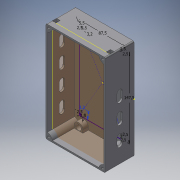
# Autodesk Inventor part: Base caixa principal
Saved by Autodesk Inventor 2019 (Build 230136000, 136)
## iProperties
Created: 2020-06-01
Part Number: Base caixa principal
Material: Generic
Document SubType Name: Modeling
Designer: luiza
Density: 1 g/cm^3
Appearance: Default
Author: luiza
Autodesk Inventor part; units mm, degrees
ref_plane "YZ Plane" through (0, 0, 0) normal (1, 0, 0) x (0, 1, 0)
ref_plane "XZ Plane" through (0, 0, 0) normal (0, 1, 0) x (-1, 0, 0)
ref_plane "XY Plane" through (0, 0, 0) normal (0, 0, 1) x (1, 0, 0)
sketch "Sketch1" plane through (0, 0, 0) normal (0, 0, 1) x (1, 0, 0)
  line L0 (-55, -92.5) -> (55, -92.5)
  line L1 (55, -92.5) -> (55, 92.5)
  line L2 (55, 92.5) -> (-55, 92.5)
  line L3 (-55, 92.5) -> (-55, -92.5)
  line L4 (-55, -92.5) -> (55, 92.5) construction
  line L5 (55, -92.5) -> (-55, 92.5) construction
  point P0 (0, 0)
  dimension "d0" = 185
  dimension "d1" = 110
  constraints: 12 end point, 2 midpoint, 2 parallel, 1 horizontal, 1 perpendicular
  measures "d0" distance of L0.end L1.end
  measures "d1" distance of L1.end L2.end
extrude "Extrusion1" add sketch "Sketch1" along normal blind 3
sketch "Sketch10" plane through (0, 0, 3) normal (0, 0, 1) x (1, 0, 0)
  line L0 (-43.75, -73.75) -> (43.75, -73.75)
  line L1 (43.75, -73.75) -> (43.75, 73.75)
  line L2 (43.75, 73.75) -> (-43.75, 73.75)
  line L3 (-43.75, 73.75) -> (-43.75, -73.75)
  line L4 (-43.75, -73.75) -> (43.75, 73.75) construction
  line L5 (43.75, -73.75) -> (-43.75, 73.75) construction
  point P0 (0, 0)
  dimension "d51" = 87.5
  dimension "d52" = 147.5
  constraints: 12 end point, 2 midpoint, 2 parallel, 1 horizontal, 1 perpendicular
  measures "d51" distance of L2.end L1.end
  measures "d52" distance of L1.end L0.end
sketch "Sketch2" plane through (0, 0, 3) normal (0, 0, 1) x (1, 0, 0)
  line L0 (-55, -92.5) -> (55, -92.5) projected
  line L1 (55, -92.5) -> (55, 92.5) projected
  line L2 (55, 92.5) -> (-55, 92.5) projected
  line L3 (-55, 92.5) -> (-55, -92.5) projected
  line L4 (56.6239, 0) -> (-62.9531, 0)
  line L5 (0, -95.1843) -> (0, 95.8224)
  line L6 (-42.8653, -89.5) -> (42.8653, -89.5)
  line L7 (52, -80.3653) -> (52, 80.3653)
  line L8 (55, 92.5) -> (-55, 92.5) projected
  arc A0 (-52, 80.3653) -> (-42.8653, 89.5) centre (-55, 92.5) ccw
  line L9 (42.8653, 89.5) -> (-42.8653, 89.5)
  line L10 (-52, 80.3653) -> (-52, -80.3653)
  arc A1 (-42.8653, -89.5) -> (-52, -80.3653) centre (-55, -92.5) ccw
  arc A2 (42.8653, 89.5) -> (52, 80.3653) centre (55, 92.5) ccw
  arc A3 (52, -80.3653) -> (42.8653, -89.5) centre (55, -92.5) ccw
  point P0 (0, 0)
  constraints: 12 end point, 9 symmetric about line, 8 point on circle, 4 centre point, 1 coincident, 1 horizontal, 1 vertical, 3 other
extrude "Extrusion2" add sketch "Sketch2" along normal blind 50 contours L3 L4 L10 A1 L6 L5 L0 | L5 L6 A3 L7 L4 L1 L0 | L3 L2 L5 L9 A0 L10 L4 | L4 L7 A2 L9 L5 L2 L1
sketch "Sketch3" plane through (0, 0, 53) normal (0, 0, 1) x (1, 0, 0)
  arc A0 (-52, 80.3653) -> (-42.8653, 89.5) centre (-55, 92.5) ccw projected
  line L0 (-42.8653, 89.5) -> (42.8653, 89.5) projected
  arc A1 (42.8653, 89.5) -> (52, 80.3653) centre (55, 92.5) ccw projected
  line L1 (52, 80.3653) -> (52, -80.3653) projected
  arc A2 (52, -80.3653) -> (42.8653, -89.5) centre (55, -92.5) ccw projected
  line L2 (42.8653, -89.5) -> (-42.8653, -89.5) projected
  arc A3 (-42.8653, -89.5) -> (-52, -80.3653) centre (-55, -92.5) ccw projected
  line L3 (-52, -80.3653) -> (-52, 80.3653) projected
  line L4 (-55, -92.5) -> (55, -92.5) projected
  line L5 (55, -92.5) -> (55, 92.5) projected
  line L6 (55, 92.5) -> (-55, 92.5) projected
  line L7 (-55, 92.5) -> (-55, -92.5) projected
  circle A4 centre (50, 87.5) radius 2.01
  line L8 (-58.744, 0) -> (58.8874, 0)
  circle A5 centre (50, -87.5) radius 2.01
  circle A6 centre (-50, 87.5) radius 2.01
  circle A7 centre (-50, -87.5) radius 2.01
  point P0 (0, 0)
  dimension "d17" = 5
  dimension "d18" = 5
  dimension "d22" = 4.02
  dimension "d57" = 5
  dimension "d58" = 5
  dimension "d59" = 5
  dimension "d60" = 5
  dimension "d61" = 5
  constraints: 4 centre point, 2 end point, 1 horizontal, 1 symmetric about line, 1 other
  measures "d17" distance from line of L5 A4.centre
  measures "d18" distance from line of L6 A4.centre
  measures "d22" diameter of A4
  measures "d57" distance from line of L7 A6.centre
  measures "d58" distance from line of L6 A6.centre
  measures "d59" distance from line of L4 A7.centre
  measures "d60" distance from line of L7 A7.centre
  measures "d61" distance from line of L4 A5.centre
extrude "Extrusion3" cut sketch "Sketch3" against normal blind 24 contours A4 | A5 | A6 | A7
ref_plane "Work Plane1" through (0, 0, 43) normal (0, 0, 1) x (1, 0, 0)
sketch "Sketch5" plane through (0, 0, 43) normal (0, 0, 1) x (1, 0, 0)
  circle A0 centre (-50, 87.5) radius 2.01 projected
  line L0 (-46.49, 92.5) -> (-46.49, 85.4735)
  line L1 (-46.49, 85.4735) -> (-50, 83.447)
  line L2 (-50, 83.447) -> (-53.51, 85.4735)
  line L3 (-53.51, 85.4735) -> (-53.51, 92.5)
  line L4 (-53.51, 89.5265) -> (-50, 91.553) construction
  line L5 (-50, 91.553) -> (-46.49, 89.5265) construction
  line L6 (55, 92.5) -> (-55, 92.5) projected
  line L7 (-46.49, 92.5) -> (-53.51, 92.5)
  line L8 (0, 97.1182) -> (0, -98.0167)
  line L9 (52.0686, 0) -> (-60.1376, 0)
  circle A1 centre (-50, -87.5) radius 2.01
  line L10 (-46.49, -92.5) -> (-46.49, -85.4735)
  line L11 (-46.49, -85.4735) -> (-50, -83.447)
  line L12 (-50, -83.447) -> (-53.51, -85.4735)
  line L13 (-53.51, -85.4735) -> (-53.51, -92.5)
  line L14 (-53.51, -89.5265) -> (-50, -91.553) construction
  line L15 (-50, -91.553) -> (-46.49, -89.5265) construction
  line L16 (-46.49, -92.5) -> (-53.51, -92.5)
  line L17 (46.49, 92.5) -> (46.49, 85.4735)
  line L18 (46.49, 85.4735) -> (50, 83.447)
  line L19 (50, 83.447) -> (53.51, 85.4735)
  line L20 (53.51, 85.4735) -> (53.51, 92.5)
  line L21 (53.51, 89.5265) -> (50, 91.553) construction
  line L22 (50, 91.553) -> (46.49, 89.5265) construction
  line L23 (46.49, 92.5) -> (53.51, 92.5)
  circle A2 centre (50, -87.5) radius 2.01
  line L24 (46.49, -92.5) -> (46.49, -85.4735)
  line L25 (46.49, -85.4735) -> (50, -83.447)
  line L26 (50, -83.447) -> (53.51, -85.4735)
  line L27 (53.51, -85.4735) -> (53.51, -92.5)
  line L28 (53.51, -89.5265) -> (50, -91.553) construction
  line L29 (50, -91.553) -> (46.49, -89.5265) construction
  line L30 (46.49, -92.5) -> (53.51, -92.5)
  line L31 (-42.8653, 89.5) -> (42.8653, 89.5) projected
  line L32 (55, -92.5) -> (55, 92.5) projected
  circle A3 centre (50, 87.5) radius 2.01 projected
  point P0 (0, 0)
  point P1 (-46.49, 87.5)
  point P2 (-46.49, -87.5)
  point P3 (46.49, 87.5)
  point P4 (46.49, -87.5)
  dimension "d54" = 7.02
  dimension "d55" = 7.02
  dimension "d56" = 7.02
  dimension "d62" = 5
  constraints: 60 end point, 29 symmetric about line, 14 point on line, 3 parallel, 2 centre point, 2 horizontal, 2 vertical, 1 equal length, 1 horizontal alignment, 1 vertical alignment, 2 other
  measures "d54" distance between parallel lines of L3 L0
  measures "d55" distance between parallel lines of L5 L2
  measures "d56" distance between parallel lines of L4 L1
  measures "d62" distance from line of L32 L18.end
extrude "Extrusion4" cut sketch "Sketch5" against normal blind 8 contours L0 L1 L2 L3 L6 | L20 L19 L18 L17 L6 | L16 L13 L12 L11 L10 | L24 L25 L26 L27 L30 | A3
fillet "Fillet1" radius 2 4 edges at (-55, 92.5, 26.5) (55, 92.5, 26.5) (-55, -92.5, 26.5) (55, -92.5, 26.5)
sketch "Sketch11" plane through (0, 0, 3) normal (0, 0, 1) x (1, 0, 0)
  circle A0 centre (-34.7653, 84.1) radius 3.01
  line L0 (-42.8653, 89.5) -> (42.8653, 89.5) projected
  circle A1 centre (-34.7653, 84.1) radius 5.1 construction
  circle A2 centre (-34.7653, 84.1) radius 8.1 construction
  line L1 (-58.7196, 0) -> (55.3155, 0)
  line L2 (0, 98.8118) -> (0, -110.7956)
  circle A3 centre (-34.7653, -84.1) radius 3.01
  circle A4 centre (34.7653, 84.1) radius 3.01
  circle A5 centre (34.7653, -84.1) radius 3.01
  arc A6 (-52, 80.3653) -> (-42.8653, 89.5) centre (-55, 92.5) ccw projected
  line L3 (-42.8653, 89.5) -> (-42.8653, 76) construction
  point P0 (0, 0)
  dimension "d63" = 6.02
  dimension "d64" = 5.4
  dimension "d65" = 10.2
  dimension "d66" = 3
  constraints: 6 centre point, 6 end point, 3 symmetric about line, 2 vertical, 1 coincident, 1 horizontal, 1 tangent, 3 other
  measures "d63" diameter of A0
  measures "d64" distance from line of L0 A0.centre
  measures "d65" diameter of A1
  measures "d66" radial gap between concentric circles of A1 A2
extrude "Extrusion7" cut sketch "Sketch11" against normal blind 3
sketch "Sketch12" plane through (0, 0, 3) normal (0, 0, 1) x (1, 0, 0)
  circle A0 centre (-34.7653, 84.1) radius 3.01 projected
  circle A1 centre (-34.7653, 84.1) radius 5.1
  arc A2 (-42.8653, 84.1) -> (-26.6653, 84.1) centre (-34.7653, 84.1) ccw
  line L0 (-26.6653, 84.1) -> (-26.6653, 92.5)
  line L1 (53, 92.5) -> (-53, 92.5) projected
  line L2 (-26.6653, 92.5) -> (-42.8653, 92.5)
  line L3 (-54.2433, 0) -> (61.8693, 0)
  line L4 (0, -98.8908) -> (0, 99.1403)
  circle A3 centre (-34.7653, -84.1) radius 5.1
  arc A4 (-26.6653, -84.1) -> (-42.8653, -84.1) centre (-34.7653, -84.1) ccw
  line L5 (-26.6653, -84.1) -> (-26.6653, -92.5)
  line L6 (-26.6653, -92.5) -> (-42.8653, -92.5)
  line L7 (-53, -92.5) -> (53, -92.5) projected
  circle A5 centre (34.7653, 84.1) radius 3.01
  circle A6 centre (34.7653, 84.1) radius 5.1
  arc A7 (26.6653, 84.1) -> (42.8653, 84.1) centre (34.7653, 84.1) ccw
  line L8 (26.6653, 84.1) -> (26.6653, 92.5)
  line L9 (26.6653, 92.5) -> (42.8653, 92.5)
  circle A8 centre (34.7653, -84.1) radius 5.1
  arc A9 (42.8653, -84.1) -> (26.6653, -84.1) centre (34.7653, -84.1) ccw
  line L10 (26.6653, -84.1) -> (26.6653, -92.5)
  line L11 (0, -92.5) -> (42.8653, -92.5)
  line L12 (42.8653, 89.5) -> (-42.8653, 89.5) projected
  line L13 (-52, -80.3653) -> (-52, 80.3653) projected
  line L14 (-42.8653, 84.1) -> (-42.8653, 92.5)
  line L15 (42.8653, 84.1) -> (42.8653, 96.4532)
  line L16 (-42.8653, -84.1) -> (-42.8653, -92.5)
  line L17 (42.8653, -84.1) -> (42.8653, -92.5)
  point P0 (0, 0)
  point P1 (-40.9253, 89.3597)
  point P2 (-40.9253, 92.5)
  point P3 (-40.9253, -92.5)
  point P4 (40.9253, 92.5)
  point P5 (40.9253, -92.5)
  dimension "d70" = 10.2
  dimension "d71" = 3
  constraints: 28 end point, 13 symmetric about line, 11 point on line, 9 centre point, 8 point on circle, 6 vertical, 2 coincident, 1 collinear, 1 horizontal, 7 other
  measures "d70" diameter of A1
  measures "d71" radial gap between concentric circles of A1 A2
extrude "Extrusion8" add sketch "Sketch12" along normal blind 10 contours L14 L12 L0 A2 | L14 L1 L0 L12 | L12 L15 A7 L8 | L8 L1 L15 L12 | L5 L6 L16 A4 | L10 A9 L17 L7
sketch "Sketch13" plane through (0, 0, 3) normal (0, 0, 1) x (1, 0, 0)
  line L0 (43.75, 73.75) -> (-43.75, 73.75) construction
  line L1 (43.75, -73.75) -> (43.75, 73.75) construction
  line L2 (-43.75, 73.75) -> (-43.75, -73.75) construction
  line L3 (-43.75, -73.75) -> (43.75, -73.75) construction
  circle A0 centre (-41.25, 71.25) radius 1.6
  line L4 (-43.4734, 71.25) -> (-34.0393, 71.25)
  line L5 (-44.5409, 71.25) -> (-42.8954, 68.4) construction
  line L6 (-42.8954, 68.4) -> (-39.6046, 68.4) construction
  line L7 (-39.6046, 68.4) -> (-37.9591, 71.25) construction
  line L8 (-37.9591, 71.25) -> (-39.6046, 74.1) construction
  line L9 (-39.6046, 74.1) -> (-42.8954, 74.1) construction
  line L10 (-42.8954, 74.1) -> (-44.5409, 71.25) construction
  line L11 (-37.8725, 77.1) -> (-34.495, 71.25)
  line L12 (-34.495, 71.25) -> (-37.8725, 65.4)
  line L13 (-37.8725, 65.4) -> (-44.6275, 65.4)
  line L14 (-44.6275, 65.4) -> (-48.005, 71.25)
  line L15 (-48.005, 71.25) -> (-44.6275, 77.1)
  line L16 (-44.6275, 77.1) -> (-37.8725, 77.1)
  line L17 (0, 102.3343) -> (0, -109.2098)
  line L18 (105.0307, 0) -> (-75.6312, 0)
  circle A1 centre (41.25, 71.25) radius 1.6
  line L19 (43.4734, 71.25) -> (34.0393, 71.25)
  line L20 (44.5409, 71.25) -> (42.8954, 68.4) construction
  line L21 (42.8954, 68.4) -> (39.6046, 68.4) construction
  line L22 (39.6046, 68.4) -> (37.9591, 71.25) construction
  line L23 (37.9591, 71.25) -> (39.6046, 74.1) construction
  line L24 (39.6046, 74.1) -> (42.8954, 74.1) construction
  line L25 (42.8954, 74.1) -> (44.5409, 71.25) construction
  line L26 (37.8725, 77.1) -> (34.495, 71.25)
  line L27 (34.495, 71.25) -> (37.8725, 65.4)
  line L28 (37.8725, 65.4) -> (44.6275, 65.4)
  line L29 (44.6275, 65.4) -> (48.005, 71.25)
  line L30 (48.005, 71.25) -> (44.6275, 77.1)
  line L31 (44.6275, 77.1) -> (37.8725, 77.1)
  circle A2 centre (-41.25, -71.25) radius 1.6
  line L32 (-43.4734, -71.25) -> (-34.0393, -71.25)
  line L33 (-44.5409, -71.25) -> (-42.8954, -68.4) construction
  line L34 (-42.8954, -68.4) -> (-39.6046, -68.4) construction
  line L35 (-39.6046, -68.4) -> (-37.9591, -71.25) construction
  line L36 (-37.9591, -71.25) -> (-39.6046, -74.1) construction
  line L37 (-39.6046, -74.1) -> (-42.8954, -74.1) construction
  line L38 (-42.8954, -74.1) -> (-44.5409, -71.25) construction
  line L39 (-37.8725, -77.1) -> (-34.495, -71.25)
  line L40 (-34.495, -71.25) -> (-37.8725, -65.4)
  line L41 (-37.8725, -65.4) -> (-44.6275, -65.4)
  line L42 (-44.6275, -65.4) -> (-48.005, -71.25)
  line L43 (-48.005, -71.25) -> (-44.6275, -77.1)
  line L44 (-44.6275, -77.1) -> (-37.8725, -77.1)
  line L45 (37.8725, -77.1) -> (34.495, -71.25)
  line L46 (37.9591, -71.25) -> (39.6046, -74.1) construction
  line L47 (39.6046, -68.4) -> (37.9591, -71.25) construction
  line L48 (34.495, -71.25) -> (37.8725, -65.4)
  line L49 (39.6046, -74.1) -> (42.8954, -74.1) construction
  circle A3 centre (41.25, -71.25) radius 1.6
  line L50 (42.8954, -74.1) -> (44.5409, -71.25) construction
  line L51 (44.6275, -77.1) -> (37.8725, -77.1)
  line L52 (42.8954, -68.4) -> (39.6046, -68.4) construction
  line L53 (44.5409, -71.25) -> (42.8954, -68.4) construction
  line L54 (37.8725, -65.4) -> (44.6275, -65.4)
  line L55 (48.005, -71.25) -> (44.6275, -77.1)
  line L56 (44.6275, -65.4) -> (48.005, -71.25)
  point P0 (0, 0)
  point P1 (-41.25, 68.4)
  point P2 (41.25, 68.4)
  point P3 (-41.25, -68.4)
  point P4 (43.4734, -71.25)
  point P5 (41.25, -68.4)
  dimension "d75" = 2.5
  dimension "d76" = 3.2
  dimension "d121" = 5.7
  dimension "d122" = 5.7
  dimension "d123" = 3
  constraints: 106 end point, 47 symmetric about line, 6 point on line, 5 equal length, 4 centre point, 4 horizontal, 1 midpoint, 1 parallel, 1 vertical, 1 vertical alignment, 8 other
  measures "d75" distance from line of L2 A0.centre
  measures "d76" diameter of A0
  measures "d121" distance between parallel lines of L7 L10
  measures "d122" distance between parallel lines of L6 L9
  measures "d123" distance between parallel lines of L8 L11
sketch "Sketch14" plane through (-55, -90.5, 0) normal (-1, 0, 0) x (0, 0, 1)
  line L0 (53, 0) -> (0, 0) projected
  line L1 (53, 181) -> (53, 0) projected
  line L2 (0, 181) -> (53, 181) projected
  line L3 (0, 181) -> (0, 0) projected
  line L4 (12.5, 19.3) -> (40.5, 19.3) construction
  line L5 (40.5, 161.7) -> (12.5, 161.7) construction
  line L6 (31.15, 137.9) -> (31.15, 149.9) construction
  line L7 (21.85, 149.9) -> (21.85, 137.9) construction
  arc A0 (21.85, 137.9) -> (31.15, 137.9) centre (26.5, 137.9) ccw construction
  arc A1 (31.15, 149.9) -> (21.85, 149.9) centre (26.5, 149.9) ccw construction
  line L8 (31.55, 149.9) -> (31.55, 137.9)
  arc A2 (21.45, 137.9) -> (31.55, 137.9) centre (26.5, 137.9) ccw
  line L9 (21.45, 137.9) -> (21.45, 149.9)
  arc A3 (31.55, 149.9) -> (21.45, 149.9) centre (26.5, 149.9) ccw
  line L10 (31.15, 102.3) -> (31.15, 114.3) construction
  line L11 (21.85, 114.3) -> (21.85, 102.3) construction
  arc A4 (21.85, 102.3) -> (31.15, 102.3) centre (26.5, 102.3) ccw construction
  arc A5 (31.15, 114.3) -> (21.85, 114.3) centre (26.5, 114.3) ccw construction
  line L12 (31.55, 114.3) -> (31.55, 102.3)
  arc A6 (21.45, 102.3) -> (31.55, 102.3) centre (26.5, 102.3) ccw
  line L13 (21.45, 102.3) -> (21.45, 114.3)
  arc A7 (31.55, 114.3) -> (21.45, 114.3) centre (26.5, 114.3) ccw
  line L14 (31.15, 66.7) -> (31.15, 78.7) construction
  line L15 (21.85, 78.7) -> (21.85, 66.7) construction
  arc A8 (21.85, 66.7) -> (31.15, 66.7) centre (26.5, 66.7) ccw construction
  arc A9 (31.15, 78.7) -> (21.85, 78.7) centre (26.5, 78.7) ccw construction
  line L16 (31.55, 78.7) -> (31.55, 66.7)
  arc A10 (21.45, 66.7) -> (31.55, 66.7) centre (26.5, 66.7) ccw
  line L17 (21.45, 66.7) -> (21.45, 78.7)
  arc A11 (31.55, 78.7) -> (21.45, 78.7) centre (26.5, 78.7) ccw
  line L18 (31.15, 31.1) -> (31.15, 43.1) construction
  line L19 (21.85, 43.1) -> (21.85, 31.1) construction
  arc A12 (21.85, 31.1) -> (31.15, 31.1) centre (26.5, 31.1) ccw construction
  arc A13 (31.15, 43.1) -> (21.85, 43.1) centre (26.5, 43.1) ccw construction
  line L20 (31.55, 43.1) -> (31.55, 31.1)
  arc A14 (21.45, 31.1) -> (31.55, 31.1) centre (26.5, 31.1) ccw
  line L21 (21.45, 31.1) -> (21.45, 43.1)
  arc A15 (31.55, 43.1) -> (21.45, 43.1) centre (26.5, 43.1) ccw
  point P0 (0, 90.5)
  point P1 (26.5, 143.9)
  point P2 (26.5, 108.3)
  point P3 (26.5, 72.7)
  point P4 (26.5, 37.1)
  point P5 (26.5, 143.9)
  point P6 (26.5, 108.3)
  point P7 (26.5, 72.7)
  point P8 (26.5, 37.1)
  dimension "d94" = 17.8
  dimension "d95" = 35.6
  dimension "d96" = 35.6
  dimension "d97" = 35.6
  dimension "d98" = 142.4
  dimension "d99" = 19.3
  dimension "d100" = 12
  dimension "d101" = 4.65
  dimension "d102" = 0.4
  dimension "d104" = 12
  dimension "d105" = 4.65
  dimension "d106" = 0.4
  dimension "d108" = 12
  dimension "d109" = 4.65
  dimension "d110" = 0.4
  dimension "d112" = 12
  dimension "d113" = 4.65
  dimension "d114" = 0.4
  constraints: 36 end point, 32 point on circle, 16 centre point, 8 parallel, 8 tangent, 12 other
  measures "d94" distance from line of point (26.5, 143.9) L5
  measures "d95" distance of point (26.5, 108.3) point (26.5, 143.9)
  measures "d96" distance of point (26.5, 72.7) point (26.5, 108.3)
  measures "d97" distance of point (26.5, 37.1) point (26.5, 72.7)
  measures "d98" distance between parallel lines of L4 L5
  measures "d99" distance between parallel lines of L2 L5
  measures "d100" distance of L6.start L6.end
  measures "d101" radius of A1
  measures "d102" distance between parallel lines of L6 L8
  measures "d104" distance of L10.start L10.end
  measures "d105" radius of A5
  measures "d106" distance between parallel lines of L10 L12
  measures "d108" distance of L14.start L14.end
  measures "d109" radius of A9
  measures "d110" distance between parallel lines of L14 L16
  measures "d112" distance of L18.start L18.end
  measures "d113" radius of A13
  measures "d114" distance between parallel lines of L18 L20
extrude "Extrusion9" cut sketch "Sketch14" against normal blind 3 contours L8 A2 L9 A3 | L12 A6 L13 A7 | L16 A10 L17 A11 | L20 A14 L21 A15
sketch "Sketch16" plane through (55, -90.5, 0) normal (1, 0, 0) x (0, 0, -1)
  arc A0 (-31.55, 66.7) -> (-21.45, 66.7) centre (-26.5, 66.7) ccw projected
  line L0 (-21.45, 78.7) -> (-21.45, 66.7) projected
  line L1 (-31.55, 66.7) -> (-31.55, 78.7) projected
  arc A1 (-21.45, 78.7) -> (-31.55, 78.7) centre (-26.5, 78.7) ccw projected
  arc A2 (-31.55, 102.3) -> (-21.45, 102.3) centre (-26.5, 102.3) ccw projected
  line L2 (-21.45, 114.3) -> (-21.45, 102.3) projected
  arc A3 (-21.45, 114.3) -> (-31.55, 114.3) centre (-26.5, 114.3) ccw projected
  line L3 (-31.55, 102.3) -> (-31.55, 114.3) projected
  arc A4 (-31.55, 31.1) -> (-21.45, 31.1) centre (-26.5, 31.1) ccw projected
  line L4 (-31.55, 31.1) -> (-31.55, 43.1) projected
  arc A5 (-21.45, 43.1) -> (-31.55, 43.1) centre (-26.5, 43.1) ccw projected
  line L5 (-21.45, 43.1) -> (-21.45, 31.1) projected
  point P0 (0, 90.5)
extrude "Extrusion10" cut sketch "Sketch16" against normal blind 3
extrude "Extrusion11" add sketch "Sketch13" along normal blind 3
sketch "Sketch17" plane through (0, 0, 6) normal (0, 0, 1) x (1, 0, 0)
  arc A0 (-38.8409, 77.1) -> (-37.5151, 76.481) centre (-34.7653, 84.1) ccw projected
  line L0 (-38.8409, 77.1) -> (-44.6275, 77.1) projected
  line L1 (-44.6275, 77.1) -> (-48.005, 71.25) projected
  line L2 (-48.005, 71.25) -> (-44.6275, 65.4) projected
  line L3 (-44.6275, 65.4) -> (-37.8725, 65.4) projected
  line L4 (-37.8725, 65.4) -> (-34.495, 71.25) projected
  line L5 (-34.495, 71.25) -> (-37.5151, 76.481) projected
  circle A1 centre (-41.25, 71.25) radius 1.6 projected
  line L6 (-44.5409, 71.25) -> (-42.8954, 74.1)
  line L7 (-42.8954, 74.1) -> (-39.6046, 74.1)
  line L8 (-39.6046, 74.1) -> (-37.9591, 71.25)
  line L9 (-37.9591, 71.25) -> (-39.6046, 68.4)
  line L10 (-39.6046, 68.4) -> (-42.8954, 68.4)
  line L11 (-42.8954, 68.4) -> (-44.5409, 71.25)
  arc A2 (37.5151, 76.481) -> (38.8409, 77.1) centre (34.7653, 84.1) ccw projected
  line L12 (37.5151, 76.481) -> (34.495, 71.25) projected
  line L13 (34.495, 71.25) -> (37.8725, 65.4) projected
  line L14 (37.8725, 65.4) -> (44.6275, 65.4) projected
  line L15 (44.6275, 65.4) -> (48.005, 71.25) projected
  line L16 (48.005, 71.25) -> (44.6275, 77.1) projected
  line L17 (44.6275, 77.1) -> (38.8409, 77.1) projected
  circle A3 centre (41.25, 71.25) radius 1.6 projected
  arc A4 (38.8409, -77.1) -> (37.5151, -76.481) centre (34.7653, -84.1) ccw projected
  line L18 (38.8409, -77.1) -> (44.6275, -77.1) projected
  line L19 (44.6275, -77.1) -> (48.005, -71.25) projected
  line L20 (48.005, -71.25) -> (44.6275, -65.4) projected
  line L21 (44.6275, -65.4) -> (37.8725, -65.4) projected
  line L22 (37.8725, -65.4) -> (34.495, -71.25) projected
  line L23 (34.495, -71.25) -> (37.5151, -76.481) projected
  circle A5 centre (41.25, -71.25) radius 1.6 projected
  arc A6 (-37.5151, -76.481) -> (-38.8409, -77.1) centre (-34.7653, -84.1) ccw projected
  line L24 (-37.5151, -76.481) -> (-34.495, -71.25) projected
  line L25 (-34.495, -71.25) -> (-37.8725, -65.4) projected
  line L26 (-37.8725, -65.4) -> (-44.6275, -65.4) projected
  line L27 (-44.6275, -65.4) -> (-48.005, -71.25) projected
  line L28 (-48.005, -71.25) -> (-44.6275, -77.1) projected
  line L29 (-44.6275, -77.1) -> (-38.8409, -77.1) projected
  circle A7 centre (-41.25, -71.25) radius 1.6 projected
  line L30 (-42.8954, -68.4) -> (-39.6046, -68.4)
  line L31 (-39.6046, -68.4) -> (-37.9591, -71.25)
  line L32 (-37.9591, -71.25) -> (-39.6046, -74.1)
  line L33 (-39.6046, -74.1) -> (-42.8954, -74.1)
  line L34 (-42.8954, -74.1) -> (-44.5409, -71.25)
  line L35 (-44.5409, -71.25) -> (-42.8954, -68.4)
  line L36 (39.6046, -68.4) -> (42.8954, -68.4)
  line L37 (42.8954, -68.4) -> (44.5409, -71.25)
  line L38 (44.5409, -71.25) -> (42.8954, -74.1)
  line L39 (42.8954, -74.1) -> (39.6046, -74.1)
  line L40 (39.6046, -74.1) -> (37.9591, -71.25)
  line L41 (37.9591, -71.25) -> (39.6046, -68.4)
  line L42 (37.9591, 71.25) -> (39.6046, 74.1)
  line L43 (39.6046, 74.1) -> (42.8954, 74.1)
  line L44 (42.8954, 74.1) -> (44.5409, 71.25)
  line L45 (44.5409, 71.25) -> (42.8954, 68.4)
  line L46 (42.8954, 68.4) -> (39.6046, 68.4)
  line L47 (39.6046, 68.4) -> (37.9591, 71.25)
  point P0 (0, 0)
  dimension "d126" = 3
  dimension "d127" = 3
  dimension "d128" = 3
  dimension "d129" = 3
  constraints: 48 end point, 20 other
  measures "d126" distance between parallel lines of L1 L6
  measures "d127" distance between parallel lines of L26 L30
  measures "d128" distance between parallel lines of L21 L36
  measures "d129" distance between parallel lines of L12 L42
extrude "Extrusion12" add sketch "Sketch17" along normal blind 3 contours A0 L5 L4 L3 L2 L1 L0 | A2 L17 L16 L15 L14 L13 L12 | A4 L23 L22 L21 L20 L19 L18 | A6 L29 L28 L27 L26 L25 L24
equation "\"d96\" = d95"
equation "\"d97\" = d95"
body "Solid1"
